Autodesk Inventor part; units mm, degrees
(part 2 of 2)
  line L405 (114.1858, -20.3362) -> (111.7265, -19.3024) construction
  spline S98 degree 3 poles (124.7413, -13.5583) (118.9615, -15.2489) (114.8814, -15.9445) (112.2229, -16.1677) knots 1.081688 1.081688 1.081688 1.081688 2 2 2 2
  line L406 (124.7413, -13.5583) -> (118.9615, -15.2489) construction
  line L407 (118.9615, -15.2489) -> (114.8814, -15.9445) construction
  line L408 (114.8814, -15.9445) -> (112.2229, -16.1677) construction
  spline S99 degree 3 poles (122.8258, -25.6525) (117.8513, -22.2585) (114.1858, -20.3362) (111.7265, -19.3024) knots 1.081688 1.081688 1.081688 1.081688 2 2 2 2
  line L409 (122.8258, -25.6525) -> (117.8513, -22.2585) construction
  line L410 (117.8513, -22.2585) -> (114.1858, -20.3362) construction
  arc A103 (124.3426, -25.8441) -> (126.2535, -13.7493) centre (0, 0) ccw
  line L411 (122.8258, -25.6525) -> (124.3426, -25.8441)
  line L412 (124.7413, -13.5583) -> (126.2535, -13.7493)
  point P0 (120.4119, -7.5757)
  point P1 (116.0628, -5.9284)
  point P2 (100.8434, 51.8265)
  point P3 (119.6986, 15.1215)
  point P4 (120.4119, 7.5757)
  point P5 (125.6092, 18.7435)
  point P6 (115.4615, 13.2043)
  point P7 (115.8906, 8.6649)
  point P8 (93.5527, 64.0569)
  point P9 (116.8596, 30.0044)
  point P10 (118.513, 22.6076)
  point P11 (122.2696, 34.3387)
  point P12 (112.8961, 27.5714)
  point P13 (113.8908, 23.1215)
  point P14 (84.7865, 75.277)
  point P15 (112.1775, 44.4142)
  point P16 (114.745, 37.2829)
  point P17 (117.0017, 49.3924)
  point P18 (108.5503, 41.5036)
  point P19 (110.0948, 37.2135)
  point P20 (74.6833, 85.31)
  point P21 (105.7264, 58.1236)
  point P22 (109.1674, 51.3703)
  point P23 (109.8886, 63.6671)
  point P24 (102.4926, 54.7813)
  point P25 (104.5626, 50.7186)
  point P26 (63.4022, 93.9976)
  point P27 (97.6079, 70.9163)
  point P28 (101.8682, 64.6475)
  point P29 (101.0425, 76.9378)
  point P30 (94.8185, 67.195)
  point P31 (97.3814, 63.4238)
  point P32 (51.1212, 101.2028)
  point P33 (87.9501, 82.5906)
  point P34 (92.9624, 76.9052)
  point P35 (90.6029, 88.9951)
  point P36 (85.649, 78.5491)
  point P37 (88.6644, 75.1288)
  point P38 (38.034, 106.812)
  point P39 (76.9052, 92.9624)
  point P40 (82.5906, 87.9501)
  point P41 (78.7344, 99.6489)
  point P42 (75.1288, 88.6644)
  point P43 (78.5491, 85.649)
  point P44 (24.347, 110.7367)
  point P45 (64.6475, 101.8682)
  point P46 (70.9163, 97.6079)
  point P47 (65.6242, 108.7311)
  point P48 (63.4238, 97.3814)
  point P49 (67.195, 94.8185)
  point P50 (10.2761, 112.915)
  point P51 (51.3703, 109.1674)
  point P52 (58.1236, 105.7264)
  point P53 (51.4791, 116.0987)
  point P54 (50.7186, 104.5626)
  point P55 (54.7813, 102.4926)
  point P56 (-3.957, 113.3125)
  point P57 (37.2829, 114.745)
  point P58 (44.4142, 112.1775)
  point P59 (36.5222, 121.6352)
  point P60 (37.2135, 110.0948)
  point P61 (41.5036, 108.5503)
  point P62 (-18.1276, 111.9231)
  point P63 (22.6076, 118.513)
  point P64 (30.0044, 116.8596)
  point P65 (20.9893, 125.2535)
  point P66 (23.1215, 113.8908)
  point P67 (27.5714, 112.8961)
  point P68 (-32.0123, 108.7685)
  point P69 (7.5757, 120.4119)
  point P70 (15.1215, 119.6986)
  point P71 (5.1253, 126.8965)
  point P72 (8.6649, 115.8906)
  point P73 (13.2043, 115.4615)
  point P74 (-45.3922, 103.8987)
  point P75 (-7.5757, 120.4119)
  point P76 (0, 120.65)
  point P77 (-10.8195, 126.5383)
  point P78 (-5.9284, 116.0628)
  point P79 (-1.371, 116.206)
  point P80 (-58.0562, 97.3902)
  point P81 (-22.6076, 118.513)
  point P82 (-15.1215, 119.6986)
  point P83 (-26.5936, 124.1845)
  point P84 (-20.4281, 114.4046)
  point P85 (-15.9246, 115.1179)
  point P86 (-69.8047, 89.3459)
  point P87 (-37.2829, 114.745)
  point P88 (-30.0044, 116.8596)
  point P89 (-41.9483, 119.8722)
  point P90 (-34.6058, 110.9421)
  point P91 (-30.2272, 112.2142)
  point P92 (-80.4523, 79.8925)
  point P93 (-51.3703, 109.1674)
  point P94 (-44.4142, 112.1775)
  point P95 (-56.6415, 113.6694)
  point P96 (-48.2376, 105.7301)
  point P97 (-44.053, 107.5409)
  point P98 (-89.8311, 69.1792)
  point P99 (-64.6475, 101.8682)
  point P100 (-58.1236, 105.7264)
  point P101 (-70.4414, 105.674)
  point P102 (-61.1087, 98.8506)
  point P103 (-57.1841, 101.1716)
  point P104 (-97.7932, 57.3749)
  point P105 (-76.9052, 92.9624)
  point P106 (-70.9163, 97.6079)
  point P107 (-83.1305, 96.0121)
  point P108 (-73.0161, 90.4122)
  point P109 (-69.4133, 93.2068)
  point P110 (-104.213, 44.6658)
  point P111 (-87.9501, 82.5906)
  point P112 (-82.5906, 87.9501)
  point P113 (-94.5085, 84.836)
  point P114 (-83.772, 80.5479)
  point P115 (-80.5479, 83.772)
  point P116 (-108.9894, 31.2522)
  point P117 (-97.6079, 70.9163)
  point P118 (-92.9624, 76.9052)
  point P119 (-104.396, 72.322)
  point P120 (-93.2068, 69.4133)
  point P121 (-90.4122, 73.0161)
  point P122 (-112.0469, 17.3458)
  point P123 (-105.7264, 58.1236)
  point P124 (-101.8682, 64.6475)
  point P125 (-112.6372, 58.6674)
  point P126 (-101.1716, 57.1841)
  point P127 (-98.8506, 61.1087)
  point P128 (-113.3374, 3.1658)
  point P129 (-112.1775, 44.4142)
  point P130 (-109.1674, 51.3703)
  point P131 (-119.102, 44.0877)
  point P132 (-107.5409, 44.053)
  point P133 (-105.7301, 48.2376)
  point P134 (-112.8405, -11.0641)
  point P135 (-116.8596, 30.0044)
  point P136 (-114.745, 37.2829)
  point P137 (-123.6885, 28.8126)
  point P138 (-112.2142, 30.2272)
  point P139 (-110.9421, 34.6058)
  point P140 (-110.564, -25.1195)
  point P141 (-119.6986, 15.1215)
  point P142 (-118.513, 22.6076)
  point P143 (-126.3243, 13.0831)
  point P144 (-115.1179, 15.9246)
  point P145 (-114.4046, 20.4281)
  point P146 (-106.5438, -38.7788)
  point P147 (-120.65, 0)
  point P148 (-120.4119, 7.5757)
  point P149 (-126.968, -2.8527)
  point P150 (-116.206, 1.371)
  point P151 (-116.0628, 5.9284)
  point P152 (-100.8434, -51.8265)
  point P153 (-119.6986, -15.1215)
  point P154 (-120.4119, -7.5757)
  point P155 (-125.6092, -18.7435)
  point P156 (-115.4615, -13.2043)
  point P157 (-115.8906, -8.6649)
  point P158 (-93.5527, -64.0569)
  point P159 (-116.8596, -30.0044)
  point P160 (-118.513, -22.6076)
  point P161 (-122.2696, -34.3387)
  point P162 (-112.8961, -27.5714)
  point P163 (-113.8908, -23.1215)
  point P164 (-84.7865, -75.277)
  point P165 (-112.1775, -44.4142)
  point P166 (-114.745, -37.2829)
  point P167 (-117.0017, -49.3924)
  point P168 (-108.5503, -41.5036)
  point P169 (-110.0948, -37.2135)
  point P170 (-74.6833, -85.31)
  point P171 (-105.7264, -58.1236)
  point P172 (-109.1674, -51.3703)
  point P173 (-109.8886, -63.6671)
  point P174 (-102.4926, -54.7813)
  point P175 (-104.5626, -50.7186)
  point P176 (-63.4022, -93.9976)
  point P177 (-97.6079, -70.9163)
  point P178 (-101.8682, -64.6475)
  point P179 (-101.0425, -76.9378)
  point P180 (-94.8185, -67.195)
  point P181 (-97.3814, -63.4238)
  point P182 (-51.1212, -101.2028)
  point P183 (-87.9501, -82.5906)
  point P184 (-92.9624, -76.9052)
  point P185 (-90.6029, -88.9951)
  point P186 (-85.649, -78.5491)
  point P187 (-88.6644, -75.1288)
  point P188 (-38.034, -106.812)
  point P189 (-76.9052, -92.9624)
  point P190 (-82.5906, -87.9501)
  point P191 (-78.7344, -99.6489)
  point P192 (-75.1288, -88.6644)
  point P193 (-78.5491, -85.649)
  point P194 (-24.347, -110.7367)
  point P195 (-64.6475, -101.8682)
  point P196 (-70.9163, -97.6079)
  point P197 (-65.6242, -108.7311)
  point P198 (-63.4238, -97.3814)
  point P199 (-67.195, -94.8185)
  dimension "d13" = 20
  dimension "d15" = 5
  dimension "d17" = 41.2647
  dimension "d18" = 9.8819
  dimension "d19" = 51.1556
  dimension "d20" = 8
  dimension "d21" = 15.7797
  dimension "d22" = 25.5016
  dimension "d23" = 1.8
  dimension "d24" = 250.952
  dimension "d27" = 360
  constraints: 256 point on circle, 226 end point, 103 centre point, 5 coincident, 4 symmetric about line, 3 horizontal, 2 perpendicular, 1 equal length, 1 horizontal alignment, 1 parallel, 1 tangent, 1803 other
  measures "d13" angle of L2 L1
  measures "d15" angle of L5 L4
  measures "d17" distance from line of L3 L0.end
  measures "d18" distance from line of L4 L3.start
  measures "d19" distance of L6.end L4.end
  measures "d20" angle of L7 L8
  measures "d21" distance from line of L3 L7.end
  measures "d22" distance of L7.end L9.end
  measures "d23" angle of L12 L11
  measures "d24" diameter of A3
extrude "Extrusion1" add sketch "Sketch1" along normal blind 3.175
sketch "Sketch2" plane through (0, 0, 0) normal (0, 1, 0) x (-1, 0, 0)
  circle A0 centre (0, 0) radius 127
  circle A1 centre (0, 0) radius 148.0058
  dimension "d31" = 254
  dimension "d32" = 296.0116
  constraints: 2 centre point, 2 coincident
  measures "d31" diameter of A0
  measures "d32" diameter of A1
extrude "Extrusion2" add sketch "Sketch2" along normal blind 3.175
sketch "Sketch3" plane through (0, 3.175, 0) normal (0, 1, 0) x (1, 0, 0)
  circle A0 centre (0, 0) radius 137.541 construction
  circle A1 centre (-137.541, 0) radius 3.175
  circle A2 centre (-68.7705, 119.114) radius 3.175
  circle A3 centre (68.7705, 119.114) radius 3.175
  circle A4 centre (137.541, 0) radius 3.175
  circle A5 centre (68.7705, -119.114) radius 3.175
  circle A6 centre (-68.7705, -119.114) radius 3.175
  dimension "d35" = 275.082
  dimension "d36" = 6.35
  dimension "d39" = 360
  constraints: 6 centre point, 1 coincident, 1 horizontal alignment, 15 other
  measures "d36" diameter of A1
extrude "Extrusion3" cut sketch "Sketch3" against normal blind 3.175
body "Solid1"
